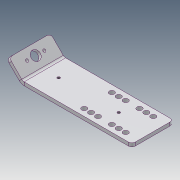
# Autodesk Inventor part: J005232
Saved by Autodesk Inventor 2015 SP1 (Build 190203100, 203)
## iProperties
Created: 2015-06-04
Material: ALUMINUM, 5052-H32
Vendor: HHMI: JRC - ID&F
Document SubType Name: Sheet Metal
Designer: ARNOLDJ
Density: 2.68 g/cm^3
Sheet Metal Rule: Default
Appearance: Metal-AL-6061 (Machined)
Part Number: J005232
Project: P-201804
Description: MBS C LED BRKT
RuleStatus: InUse
AfterDocSave0: file://Part Number Cleaner
DESIGN DEPARTMENT: HHMI: JRC - ID&F
SPECIAL FINISH: NONE
LAB/DEPT: SVOBODA (LAB)
REQUESTING SCIENTIST: SOFRONIEW, NICK
SURFACE ROUGHNESS: 63 Ra
Thickness: 0.125 in
ALTERED ITEM PART NUMBER: N/A
ALTERED ITEM VENDOR: N/A
ALTERED ITEM DESCRIPTION: N/A
Revision Number: -
Autodesk Inventor part; units mm, degrees
ref_plane "YZ Plane" through (0, 0, 0) normal (1, 0, 0) x (0, 1, 0)
ref_plane "XZ Plane" through (0, 0, 0) normal (0, 1, 0) x (-1, 0, 0)
ref_plane "XY Plane" through (0, 0, 0) normal (0, 0, 1) x (1, 0, 0)
sketch "Sketch1" plane through (0, 0, 0) normal (0, 1, 0) x (-1, 0, 0)
  line L0 (-50.8, -19.05) -> (50.8, -19.05)
  line L1 (50.8, -19.05) -> (50.8, 19.05)
  line L2 (50.8, 19.05) -> (-50.8, 19.05)
  line L3 (-50.8, 19.05) -> (-50.8, -19.05)
  line L4 (-50.8, -19.05) -> (50.8, 19.05) construction
  line L5 (50.8, -19.05) -> (-50.8, 19.05) construction
  point P0 (0, 0)
  dimension "d0" = 38.1
  dimension "d1" = 101.6
  measures "d0" distance of L0.end L1.end
  measures "d1" distance of L1.end L2.end
extrude "Plate1" add sketch "Sketch1" along normal blind 3.175
sketch "Sketch2" plane through (-48.5549, 2.2451, 19.05) normal (-0.7071068, -0.7071068, 0) x (0.7071068, -0.7071068, 0)
  line L0 (0, -38.1) -> (0, 0)
  line L1 (0, 0) -> (-19.05, 0)
  line L2 (-19.05, 0) -> (-19.05, -38.1)
  line L3 (-19.05, -38.1) -> (0, -38.1)
  constraints: 6 end point, 1 horizontal, 1 perpendicular, 1 vertical
edge flange "Flange1" height 19.05 angle 45 thickness 3.175 bend radius 3.175 thickness toward (-0.7071068, -0.7071068, 0) relief tear relief width 3.175 relief depth 1.5875 edges at (-50.8, 3.175, 0) wall of the first edge with corners at (-48.5549, 2.2451, -19.05) (-48.5549, 2.2451, 19.05) (-62.0253, 15.7154, 19.05) (-62.0253, 15.7154, -19.05)
bend "Bend1"
corner "Corner1"
sketch "Sketch3" plane through (-62.0253, 15.7154, -19.05) normal (0.7071068, 0.7071068, 0) x (-0.7071068, 0.7071068, 0)
  circle A0 centre (-7.62, 19.05) radius 4.1275
  circle A1 centre (-7.62, 26.9875) radius 1.2446
  circle A2 centre (-7.62, 11.1125) radius 1.2446
  line L0 (-132.4339, 19.05) -> (42.7893, 19.05) projected
  line L1 (0, 0) -> (0, 38.1) projected
  point P0 (-54.971, 19.05)
  dimension "d13" = 8.255
  dimension "d14" = 2.4892
  dimension "d15" = 7.9375
  dimension "d16" = 7.9375
  dimension "d17" = 7.62
  constraints: 3 centre point, 2 vertical alignment, 1 equal radius, 1 point on line
  measures "d13" diameter of A0
  measures "d14" diameter of A1
  measures "d15" distance of A0.centre A1.centre
  measures "d16" distance of A2.centre A0.centre
  measures "d17" distance from line of A0.centre L1
extrude "Cut1" cut sketch "Sketch3" against normal blind 3.175
sketch "Sketch4" plane through (0, 3.175, 0) normal (0, 1, 0) x (1, 0, 0)
  line L0 (32.385, -12.7) -> (6.985, -12.7)
  line L1 (6.985, -12.7) -> (6.985, 12.7)
  line L2 (6.985, 12.7) -> (32.385, 12.7)
  line L3 (32.385, 12.7) -> (32.385, -12.7)
  line L4 (32.385, -12.7) -> (6.985, 12.7) construction
  line L5 (6.985, -12.7) -> (32.385, 12.7) construction
  line L6 (50.8, 19.05) -> (50.8, -19.05) projected
  point P0 (0, 0)
  point P1 (19.685, 0)
  point P2 (32.385, -12.7)
  point P3 (38.735, -12.7)
  point P4 (26.035, -12.7)
  point P5 (13.335, -12.7)
  point P6 (0.635, -12.7)
  point P7 (13.335, 12.7)
  point P8 (0.635, 12.7)
  point P9 (26.035, 12.7)
  point P10 (38.735, 12.7)
  point P11 (-35.56, 0)
  point P12 (19.685, 0)
  point P13 (19.685, 0)
  dimension "d20" = 25.4
  dimension "d21" = 25.4
  dimension "d32" = 19.685
  dimension "d33" = 6.35
  dimension "d34" = 6.35
  dimension "d35" = 6.35
  dimension "d36" = 6.35
  dimension "d37" = 35.56
  constraints: 12 end point, 5 coincident, 5 point on line, 4 vertical alignment, 3 midpoint, 2 parallel, 1 horizontal, 1 perpendicular
  measures "d20" distance of L2.end L0.start
  measures "d21" distance of L1.end L2.end
  measures "d32" distance of point (19.685, 0) point (0, 0)
  measures "d33" distance of point (32.385, -12.7) point (38.735, -12.7)
  measures "d34" distance of point (32.385, -12.7) point (26.035, -12.7)
  measures "d35" distance of point (6.985, -12.7) point (0.635, -12.7)
  measures "d36" distance of point (6.985, -12.7) point (13.335, -12.7)
  measures "d37" distance of point (-35.56, 0) point (0, 0)
hole "Hole1" at (6.985, 3.175, -12.7) at (32.385, 3.175, -12.7) at (32.385, 3.175, 12.7) at (6.985, 3.175, 12.7) at (38.735, 3.175, 12.7) at (26.035, 3.175, 12.7) at (38.735, 3.175, -12.7) at (13.335, 3.175, -12.7) at (26.035, 3.175, -12.7) at (0.635, 3.175, -12.7) at (0.635, 3.175, 12.7) at (13.335, 3.175, 12.7) direction (0, -1, 0) diameter 4.7625 depth 3.175 tip angle 118
fillet "Corner Round1" radius 3.175 4 edges at (-63.1479, 14.5929, -19.05) (-63.1479, 14.5929, 19.05) (50.8, 1.5875, -19.05) (50.8, 1.5875, 19.05)
sketch "Sketch5" plane through (0, 0, 0) normal (0, 0, 1) x (1, 0, 0)
  line L0 (-104.5658, 0) -> (17.4276, 0) projected
  line L1 (17.4757, 84.4402) -> (-106.4259, -39.4614) projected
  line L2 (-52.6599, 1.8599) -> (-62.0253, 11.2253) projected
  line L3 (-58.8822, 8.0822) -> (-90.3131, -23.3487)
  point P0 (0, 0)
  dimension "d31" = 44.45
  constraints: 3 point on line, 2 end point
  measures "d31" distance of L3.start L3.end
hole "Hole2" at (-35.56, 3.175, 0) at (19.685, 3.175, 0) direction (0, -1, 0) diameter 2.4638 end through all
equation "\"d18\" = Thickness"
equation "\"d28\" = Thickness"
equation "\"d3\" = BendReliefWidth"
equation "\"d4\" = BendReliefDepth"
equation "\"d5\" = MinimumRemnant"
equation "\"d6\" = BendRadius"
equation "\"d9\" = BendRadius"
equation "\"d10\" = CornerReliefSize"
equation "\"d11\" = GapSize"
equation "\"d12\" = JacobiRadiusSize"
equation "\"BendRadius\" = Thickness"
equation "\"BendReliefWidth\" = Thickness"
equation "\"BendReliefDepth\" = 0.5 * Thickness"
equation "\"CornerReliefSize\" = 4 * Thickness"
equation "\"MinimumRemnant\" = 2 * Thickness"
equation "\"TransitionRadius\" = BendRadius"
equation "\"JacobiRadiusSize\" = BendRadius"
equation "\"GapSize\" = Thickness"
equation "\"d2\" = BendRadius"
equation "\"Thickness\" = 3.175"
body "Solid1"
